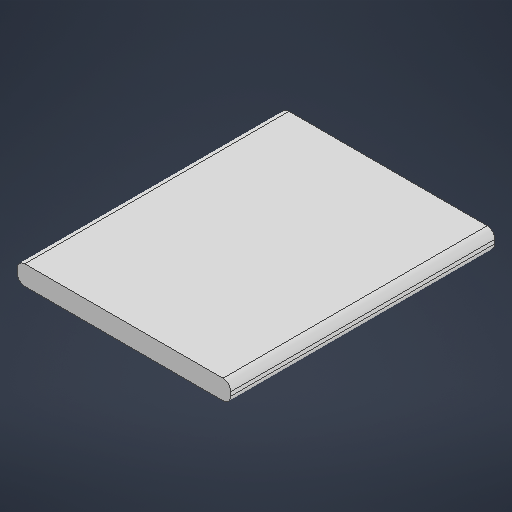
# Autodesk Inventor part: Battery_prop
Saved by Autodesk Inventor 2026.2 (Build 302298010, 298A)
## iProperties
Created: 2026-09-18
Part Number: Battery_prop
Material: Ogólny
Document SubType Name: Modeling
Designer: Rozkurwiator
Density: 1 g/cm^3
Appearance: Domyślna
Author: Rozkurwiator
Autodesk Inventor part; units mm, degrees
ref_plane "YZ Plane" through (0, 0, 0) normal (1, 0, 0) x (0, 1, 0)
ref_plane "XZ Plane" through (0, 0, 0) normal (0, 1, 0) x (-1, 0, 0)
ref_plane "XY Plane" through (0, 0, 0) normal (0, 0, 1) x (1, 0, 0)
sketch "Szkic1" plane through (0, 0, 0) normal (0, 1, 0) x (-1, 0, 0)
  line L0 (-27.5, 34) -> (27.5, 34)
  line L1 (27.5, 34) -> (27.5, -34)
  line L2 (27.5, -34) -> (-27.5, -34)
  line L3 (-27.5, -34) -> (-27.5, 34)
  line L4 (-27.5, 34) -> (27.5, -34) construction
  line L5 (27.5, 34) -> (-27.5, -34) construction
  point P0 (0, 0)
  dimension "d0" = 55
  dimension "d1" = 68
  constraints: 12 end point, 2 midpoint, 2 parallel, 1 horizontal, 1 perpendicular
  measures "d0" distance of L1.end L2.end
  measures "d1" distance of L0.end L1.end
extrude "Wyciągnięcie proste1" add sketch "Szkic1" along normal blind 5
fillet "Zaokrąglenie1" radius 2 4 edges at (27.5, 5, 0) (27.5, 0, 0) (-27.5, 0, 0) (-27.5, 5, 0)
